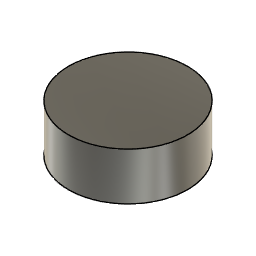
New_Gear_Assembly v14 (Autodesk Fusion 360 archive; units mm, degrees)
design "diametric magnet"
Autodesk Fusion 360 part; units mm, degrees
sketch "Sketch1" plane through (0, 0, 0) normal (0, 0, 1) x (1, 0, 0)
  circle A0 centre (0, 0) radius 3.9751
  dimension "d1" = 7.9502
  constraint coincident A0.centre origin
  measures "d1" diameter of A0
extrude "Extrude1" add sketch "Sketch1" along normal blind 3.175

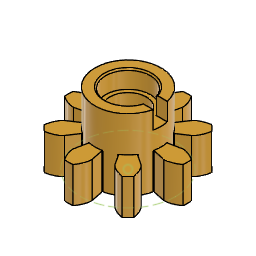
design "Spur Gear (8 teeth)"
description: Spur Gear; Diametrial Pitch: 12.0; Num Teeth: 8; Pressure Angle: 14.500000000000002; Backlash: 0.00 in
Autodesk Fusion 360 part; units mm, degrees
sketch "Sketch1" plane through (0, 0, 0) normal (0, 0, 1) x (1, 0, 0)
  circle A0 centre (0, 0) radius 5.8759
  circle A1 centre (0, 0) radius 1.75
extrude "Extrude1" add sketch "Sketch1" along normal blind 6.35
sketch "Sketch2" plane through (0, 0, 0) normal (0, 0, 1) x (1, 0, 0)
  spline S0 degree 5 poles (8.0305, -1.6437) (8.0375, -1.6451) (8.0514, -1.6477) (8.0725, -1.6509) (8.1008, -1.6537) (8.1364, -1.6553) (8.1722, -1.6555) (8.2081, -1.6549) (8.2441, -1.6538) (8.2802, -1.6524) (8.3163, -1.6506) (8.3525, -1.6484) (8.3887, -1.6456) (8.425, -1.6421) (8.4614, -1.6378) (8.4979, -1.633) (8.5343, -1.6276) (8.5709, -1.6217) (8.6074, -1.6154) (8.644, -1.6088) (8.6806, -1.6017) (8.7172, -1.5942) (8.7538, -1.5863) (8.7904, -1.5779) (8.8271, -1.5691) (8.8638, -1.5599) (8.9004, -1.5502) (8.9371, -1.5402) (8.9738, -1.5298) (9.0105, -1.519) (9.0471, -1.5078) (9.0838, -1.4963) (9.1205, -1.4844) (9.1571, -1.4721) (9.1937, -1.4595) (9.2304, -1.4465) (9.267, -1.4332) (9.3035, -1.4195) (9.3401, -1.4055) (9.3766, -1.3911) (9.4132, -1.3764) (9.4496, -1.3613) (9.4861, -1.346) (9.5225, -1.3303) (9.5589, -1.3142) (9.5953, -1.2978) (9.6316, -1.2812) (9.6678, -1.2642) (9.7041, -1.2468) (9.7403, -1.2292) (9.7764, -1.2112) (9.8125, -1.193) (9.8486, -1.1744) (9.8846, -1.1555) (9.9206, -1.1363) (9.9565, -1.1168) (9.9923, -1.097) (10.0281, -1.0769) (10.0639, -1.0565) (10.0996, -1.0358) (10.1352, -1.0149) (10.1707, -0.9936) (10.2062, -0.972) (10.2417, -0.9502) (10.277, -0.928) (10.3123, -0.9056) (10.3476, -0.8829) (10.3827, -0.8599) (10.4178, -0.8366) (10.4528, -0.813) (10.4878, -0.7892) (10.5156, -0.7699) (10.5365, -0.7553) (10.5504, -0.7455) (10.5574, -0.7406) knots 0 0 0 0 0 0 0.01428571 0.02857143 0.04285714 0.05714286 0.07142857 0.08571429 0.1 0.11428571 0.12857143 0.14285714 0.15714286 0.17142857 0.18571429 0.2 0.21428571 0.22857143 0.24285714 0.25714286 0.27142857 0.28571429 0.3 0.31428571 0.32857143 0.34285714 0.35714286 0.37142857 0.38571429 0.4 0.41428571 0.42857143 0.44285714 0.45714286 0.47142857 0.48571429 0.5 0.51428571 0.52857143 0.54285714 0.55714286 0.57142857 0.58571429 0.6 0.61428571 0.62857143 0.64285714 0.65714286 0.67142857 0.68571429 0.7 0.71428571 0.72857143 0.74285714 0.75714286 0.77142857 0.78571429 0.8 0.81428571 0.82857143 0.84285714 0.85714286 0.87142857 0.88571429 0.9 0.91428571 0.92857143 0.94285714 0.95714286 0.97142857 0.98571429 1 1 1 1 1 1
  spline S1 degree 5 poles (8.0305, 1.6437) (8.0375, 1.6451) (8.0514, 1.6477) (8.0725, 1.6509) (8.1008, 1.6537) (8.1364, 1.6553) (8.1722, 1.6555) (8.2081, 1.6549) (8.2441, 1.6538) (8.2802, 1.6524) (8.3163, 1.6506) (8.3525, 1.6484) (8.3887, 1.6456) (8.425, 1.6421) (8.4614, 1.6378) (8.4979, 1.633) (8.5343, 1.6276) (8.5709, 1.6217) (8.6074, 1.6154) (8.644, 1.6088) (8.6806, 1.6017) (8.7172, 1.5942) (8.7538, 1.5863) (8.7904, 1.5779) (8.8271, 1.5691) (8.8638, 1.5599) (8.9004, 1.5502) (8.9371, 1.5402) (8.9738, 1.5298) (9.0105, 1.519) (9.0471, 1.5078) (9.0838, 1.4963) (9.1205, 1.4844) (9.1571, 1.4721) (9.1937, 1.4595) (9.2304, 1.4465) (9.267, 1.4332) (9.3035, 1.4195) (9.3401, 1.4055) (9.3766, 1.3911) (9.4132, 1.3764) (9.4496, 1.3613) (9.4861, 1.346) (9.5225, 1.3303) (9.5589, 1.3142) (9.5953, 1.2978) (9.6316, 1.2812) (9.6678, 1.2642) (9.7041, 1.2468) (9.7403, 1.2292) (9.7764, 1.2112) (9.8125, 1.193) (9.8486, 1.1744) (9.8846, 1.1555) (9.9206, 1.1363) (9.9565, 1.1168) (9.9923, 1.097) (10.0281, 1.0769) (10.0639, 1.0565) (10.0996, 1.0358) (10.1352, 1.0149) (10.1707, 0.9936) (10.2062, 0.972) (10.2417, 0.9502) (10.277, 0.928) (10.3123, 0.9056) (10.3476, 0.8829) (10.3827, 0.8599) (10.4178, 0.8366) (10.4528, 0.813) (10.4878, 0.7892) (10.5156, 0.7699) (10.5365, 0.7553) (10.5504, 0.7455) (10.5574, 0.7406) knots 0 0 0 0 0 0 0.01428571 0.02857143 0.04285714 0.05714286 0.07142857 0.08571429 0.1 0.11428571 0.12857143 0.14285714 0.15714286 0.17142857 0.18571429 0.2 0.21428571 0.22857143 0.24285714 0.25714286 0.27142857 0.28571429 0.3 0.31428571 0.32857143 0.34285714 0.35714286 0.37142857 0.38571429 0.4 0.41428571 0.42857143 0.44285714 0.45714286 0.47142857 0.48571429 0.5 0.51428571 0.52857143 0.54285714 0.55714286 0.57142857 0.58571429 0.6 0.61428571 0.62857143 0.64285714 0.65714286 0.67142857 0.68571429 0.7 0.71428571 0.72857143 0.74285714 0.75714286 0.77142857 0.78571429 0.8 0.81428571 0.82857143 0.84285714 0.85714286 0.87142857 0.88571429 0.9 0.91428571 0.92857143 0.94285714 0.95714286 0.97142857 0.98571429 1 1 1 1 1 1
  arc A0 (10.5574, -0.7406) -> (10.5574, 0.7406) centre (0, 0) ccw
  line L0 (5.7467, -1.1783) -> (8.0305, -1.6437)
  line L1 (5.7467, 1.1783) -> (8.0305, 1.6437)
  line L2 (5.7467, -1.1783) -> (5.7467, 1.1783)
  point P0 (8.2021, -1.6549)
  point P1 (8.3777, -1.6463)
  point P2 (8.5556, -1.6241)
  point P3 (8.7352, -1.5903)
  point P4 (8.9162, -1.5458)
  point P5 (9.0983, -1.4916)
  point P6 (9.281, -1.4279)
  point P7 (9.4641, -1.3552)
  point P8 (9.6473, -1.2737)
  point P9 (9.8305, -1.1837)
  point P10 (10.0133, -1.0852)
  point P11 (10.1956, -0.9784)
  point P12 (10.377, -0.8635)
  point P13 (8.2021, 1.6549)
  point P14 (8.3777, 1.6463)
  point P15 (8.5556, 1.6241)
  point P16 (8.7352, 1.5903)
  point P17 (8.9162, 1.5458)
  point P18 (9.0983, 1.4916)
  point P19 (9.281, 1.4279)
  point P20 (9.4641, 1.3552)
  point P21 (9.6473, 1.2737)
  point P22 (9.8305, 1.1837)
  point P23 (10.0133, 1.0852)
  point P24 (10.1956, 0.9784)
  point P25 (10.377, 0.8635)
extrude "Extrude2" add sketch "Sketch2" along normal blind 6.35
fillet "Fillet1" radius 0.1016 2 edges at (5.7561, -1.1802, 3.175) (5.7561, 1.1802, 3.175)
pattern_circular "C-Pattern1" count 8 over 360 about axis through (0, 0, 0) along (0, 0, 1) of "Extrude2", "Fillet1"
sketch "Sketch3" plane through (0, 0, 0) normal (0, 0, 1) x (1, 0, 0)
  circle A0 centre (0, 0) radius 8.4667 construction
sketch "sketch 835" plane through (0, 0, 6.35) normal (0, 0, 1) x (-1, 0, 0)
  circle A0 centre (0, 0) radius 6.35
extrude "Extrude3" add sketch "sketch 835" along normal blind 6.35
hole "Hole1" at (0, 0, 12.7) direction (0, 0, -1) diameter 3.4036 depth 17.78 tip angle 118 counterbore diameter 6.5024 counterbore depth 2.9972
extrude "Extrude5" cut 1 faces at (0.2461, -2.7163, 9.7028) along direction (0, 0, -1) blind 5.08
sketch "sketch 848" plane through (0, 0, 12.7) normal (0, 0, 1) x (-1, 0, 0)
  circle A0 centre (0, 0) radius 3.9688
extrude "Extrude4" cut sketch "sketch 848" against normal blind 3.175
sketch "Sketch4" plane through (0, 0, 12.7) normal (0, 0, 1) x (-1, 0, 0)
  circle A0 centre (0, 0) radius 6.35
  arc A1 (-5.7353, -1.2777) -> (-4.9589, -3.1519) centre (0, 0) ccw
  arc A2 (-5.7353, -1.2777) -> (-4.9589, -3.1519) centre (0, 0) ccw
  circle A3 centre (0, 0) radius 5.8759
  constraint concentric A0 A3
  constraint coincident A1.end A3
extrude "Extrude6" cut sketch "Sketch4" against normal blind 6.35
chamfer "Chamfer1" distance 0.254 angle 45 1 edges at (3.7002, -1.4352, 12.7)
sketch "Sketch5" plane through (0, 0, 12.7) normal (0, 0, 1) x (-1, 0, 0)
  line L0 (-3.307, -1.27) -> (-6.635, -1.27)
  line L1 (-6.635, -1.27) -> (-6.635, 1.27)
  line L2 (-6.635, 1.27) -> (-3.307, 1.27)
  line L3 (-3.307, 1.27) -> (-3.307, -1.27)
  line L4 (0, 0) -> (-3.307, 0)
  dimension "d4" = 2.54
  constraint horizontal L0
  constraint vertical L1
  constraint horizontal L2
  constraint vertical L3
  constraint coincident L4.start origin
  constraint midpoint L3 L4.end
  constraint horizontal L4
  measures "d4" distance of L0.end L1.end
extrude "Extrude7" cut sketch "Sketch5" against normal up to surface (3.175 mm away)
